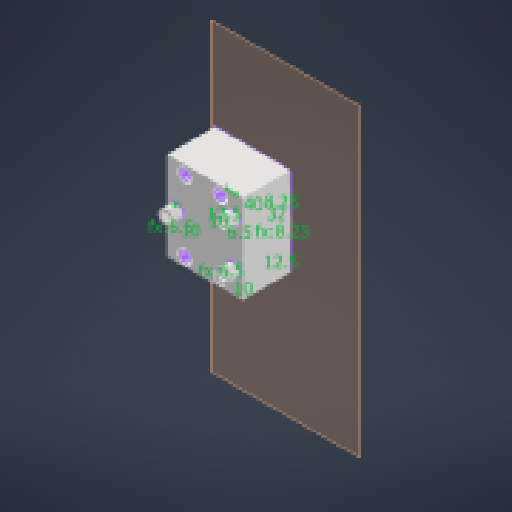
# Autodesk Inventor part: Printer_head_mount
Saved by Autodesk Inventor 2027 (Build 310192060, 192F)
## iProperties
Created: 2026-06-01
Part Number: Printer_head_mount
Material: Generic
Document SubType Name: Modeling
Designer: jacob
Density: 1 g/cm^3
Appearance: Default
Author: jacob
Autodesk Inventor part; units mm, degrees
ref_plane "YZ Plane" through (0, 0, 0) normal (1, 0, 0) x (0, 1, 0)
ref_plane "XZ Plane" through (0, 0, 0) normal (0, 1, 0) x (-1, 0, 0)
ref_plane "XY Plane" through (0, 0, 0) normal (0, 0, 1) x (1, 0, 0)
ref_plane "Work Plane1" through (0, 0, 0) normal (0, 0, 1) x (1, 0, 0)
sketch "base_sketch" plane through (0, 0, 0) normal (0, 0, 1) x (1, 0, 0)
  line L0 (3.4991, 43.75) -> (-50, 43.75)
  line L1 (-50, 43.75) -> (-50, -18.8295)
  line L2 (-50, -18.8295) -> (3.4991, -18.8295)
  line L3 (3.4991, -18.8295) -> (3.4991, 43.75)
  line L4 (-37.5, -12.5795) -> (-37.5, -18.8295)
  line L5 (-37.5, -12.5795) -> (-50, -12.5795)
  line L6 (3.4991, -12.3536) -> (-9, -12.5)
  line L7 (-2.7504, -12.4268) -> (-2.7504, -3.4634)
  line L8 (-2.7504, -3.4634) -> (-2.7504, -11.9897)
  line L9 (-2.7504, 37.5) -> (-2.7504, 28.5366)
  line L10 (-2.791, 23.7736) -> (-6.8956, 26.1903)
  line L11 (-6.8956, 26.1903) -> (-6.855, 30.9533)
  line L12 (-6.855, 30.9533) -> (-2.7098, 33.2996)
  line L13 (-2.7098, 33.2996) -> (1.3947, 30.8829)
  line L14 (1.3947, 30.8829) -> (1.3541, 26.12)
  line L15 (1.3541, 26.12) -> (-2.791, 23.7736)
  line L16 (-2.762, 1.2997) -> (1.3688, -1.0718)
  line L17 (1.3688, -1.0718) -> (1.3804, -5.8349)
  line L18 (1.3804, -5.8349) -> (-2.7388, -8.2265)
  line L19 (-2.7388, -8.2265) -> (-6.8696, -5.855)
  line L20 (-6.8696, -5.855) -> (-6.8812, -1.0919)
  line L21 (-6.8812, -1.0919) -> (-2.762, 1.2997)
  line L22 (-2.7504, 28.5366) -> (-2.7504, -3.4634)
  line L23 (-2.7504, -3.4634) -> (-2.7504, 12.5366)
  line L24 (-2.7504, 12.5366) -> (-42.7504, 12.5366)
  line L25 (-42.7504, 7.7735) -> (-46.8754, 10.155)
  line L26 (-46.8754, 10.155) -> (-46.8754, 14.9182)
  line L27 (-46.8754, 14.9182) -> (-42.7504, 17.2998)
  line L28 (-42.7504, 17.2998) -> (-38.6254, 14.9182)
  line L29 (-38.6254, 14.9182) -> (-38.6254, 10.155)
  line L30 (-38.6254, 10.155) -> (-42.7504, 7.7735)
  dimension "d20" = 12.5
  dimension "d26" = 12.5
  dimension "d29" = 32
  dimension "d30" = 8.25
  dimension "d31" = 8.25
  dimension "d32" = 40
  constraints: 62 end point, 4 perpendicular, 4 point on line, 3 coincident, 3 vertical, 2 midpoint, 2 parallel, 1 collinear, 1 horizontal, 39 other
  measures "d20" distance of L4.start L5.end
  measures "d26" distance of L6.start L6.end
  measures "d29" distance of L7.end L9.end
  measures "d30" distance between parallel lines of L11 L14
  measures "d31" distance between parallel lines of L20 L17
  measures "d32" distance of L23.end L24.end
extrude "first" add sketch "base_sketch" along normal blind 20
sketch "Sketch6" plane through (0, 0, 20) normal (0, 0, 1) x (1, 0, 0)
  line L0 (3.4991, 43.75) -> (-50, 43.75) projected
  line L1 (-50, 43.75) -> (-50, -18.8295) projected
  line L2 (-50, -18.8295) -> (3.4991, -18.8295) projected
  line L3 (3.4991, -18.8295) -> (3.4991, 43.75) projected
  line L4 (-38.6254, 14.9182) -> (-38.6254, 10.155) projected
  line L5 (-38.6254, 10.155) -> (-42.7504, 7.7735) projected
  line L6 (-42.7504, 7.7735) -> (-46.8754, 10.155) projected
  line L7 (-46.8754, 10.155) -> (-46.8754, 14.9182) projected
  line L8 (-46.8754, 14.9182) -> (-42.7504, 17.2998) projected
  line L9 (-42.7504, 17.2998) -> (-38.6254, 14.9182) projected
  line L10 (1.3541, 26.12) -> (-2.791, 23.7736) projected
  line L11 (-2.791, 23.7736) -> (-6.8956, 26.1903) projected
  line L12 (-6.8956, 26.1903) -> (-6.855, 30.9533) projected
  line L13 (-6.855, 30.9533) -> (-2.7098, 33.2996) projected
  line L14 (-2.7098, 33.2996) -> (1.3947, 30.8829) projected
  line L15 (1.3947, 30.8829) -> (1.3541, 26.12) projected
  line L16 (-2.762, 1.2997) -> (1.3688, -1.0718) projected
  line L17 (1.3688, -1.0718) -> (1.3804, -5.8349) projected
  line L18 (1.3804, -5.8349) -> (-2.7388, -8.2265) projected
  line L19 (-2.7388, -8.2265) -> (-6.8696, -5.855) projected
  line L20 (-6.8696, -5.855) -> (-6.8812, -1.0919) projected
  line L21 (-6.8812, -1.0919) -> (-2.762, 1.2997) projected
  circle A0 centre (-12.5, 37.5) radius 3.25 projected
  point P0 (0, 0)
extrude "middle" add sketch "Sketch6" along normal blind 7 from surface at 0
sketch "Sketch7" plane through (0, 0, 27) normal (0, 0, 1) x (1, 0, 0)
  line L0 (-50, 43.75) -> (-50, -18.8295) projected
  line L1 (-50, -18.8295) -> (3.4991, -18.8295) projected
  line L2 (3.4991, -18.8295) -> (3.4991, 43.75) projected
  line L3 (3.4991, 43.75) -> (-50, 43.75) projected
  circle A0 centre (-12.25, -12.5) radius 3.25 projected
  circle A1 centre (-37.5, 37.5) radius 3.25 projected
  circle A2 centre (-37.5, -12.5795) radius 3.25 projected
  point P0 (0, 0)
extrude "top" add sketch "Sketch7" along normal blind 7 contours L3 L2 L1 L0 | A0 | A1 | A2
sketch "standoffs" plane through (0, 0, 34) normal (0, 0, 1) x (1, 0, 0)
  circle A0 centre (-3.0004, 28.5366) radius 3.25
  circle A1 centre (-3.0004, -3.4634) radius 3.25
  circle A2 centre (-43.0004, 12.5366) radius 3.25
  circle A3 centre (-3.0004, 28.5366) radius 5
  circle A4 centre (-3.0004, -3.4634) radius 5
  circle A5 centre (-43.0004, 12.5366) radius 5
  dimension "d54" = 10
  dimension "d55" = 10
  dimension "d56" = 10
  dimension "d61" = 6.5
  dimension "d62" = 6.5
  dimension "d63" = 6.5
  constraints: 6 centre point, 3 coincident
  measures "d54" diameter of A3
  measures "d55" diameter of A4
  measures "d56" diameter of A5
  measures "d61" diameter of A0
  measures "d62" diameter of A1
  measures "d63" diameter of A2
extrude "Extrusion7" add sketch "standoffs" along normal blind 8
sketch "label_sketch" plane through (-50, -18.8295, 0) normal (-1, 0, 0) x (0, 0, 1)
  line L0 (21.8439, 46.335) -> (21.8439, 9.2504) construction
  line L1 (21.8439, 9.2504) -> (5.5419, 9.2504) construction
  line L2 (5.5419, 9.2504) -> (5.5419, 46.335) construction
  line L3 (5.5419, 46.335) -> (21.8439, 46.335) construction
  spline S0 degree 2 poles (20.7892, 44.0996) (20.5916, 44.0996) (20.2359, 44.2404) (20.1124, 44.3664) knots 0 0 0 1 2 2 2
  spline S1 degree 2 poles (20.1124, 44.3664) (19.9568, 44.5244) (19.7963, 44.9518) (19.7963, 45.2778) knots 0 0 0 1 2 2 2
  line L4 (19.7963, 45.2778) -> (19.7963, 45.6211)
  line L5 (19.7963, 45.6211) -> (18.6601, 45.6211)
  line L6 (18.6601, 45.6211) -> (18.6601, 46.0262)
  line L7 (18.6601, 46.0262) -> (21.7081, 46.0262)
  line L8 (21.7081, 46.0262) -> (21.7081, 45.2605)
  spline S2 degree 2 poles (21.7081, 45.2605) (21.7081, 44.9888) (21.6191, 44.6084) (21.5179, 44.4627) knots 0 0 0 1 2 2 2
  spline S3 degree 2 poles (21.5179, 44.4627) (21.4018, 44.2923) (21.0436, 44.0996) (20.7892, 44.0996) knots 0 0 0 1 2 2 2
  spline S4 degree 2 poles (20.7769, 44.522) (20.9349, 44.522) (21.1671, 44.6307) (21.2412, 44.7418) knots 0 0 0 1 2 2 2
  spline S5 degree 2 poles (21.2412, 44.7418) (21.3055, 44.8381) (21.3573, 45.095) (21.3573, 45.2852) knots 0 0 0 1 2 2 2
  line L9 (21.3573, 45.2852) -> (21.3573, 45.6211)
  line L10 (21.3573, 45.6211) -> (20.1421, 45.6211)
  line L11 (20.1421, 45.6211) -> (20.1421, 45.3445)
  spline S6 degree 2 poles (20.1421, 45.3445) (20.1421, 45.0975) (20.2211, 44.7937) (20.3249, 44.6949) knots 0 0 0 1 2 2 2
  spline S7 degree 2 poles (20.3249, 44.6949) (20.4162, 44.6035) (20.6311, 44.522) (20.7769, 44.522) knots 0 0 0 1 2 2 2
  line L12 (20.5348, 42.5311) -> (20.5348, 42.5509)
  spline S8 degree 2 poles (20.5348, 42.5509) (20.5472, 42.5954) (20.5521, 42.6917) (20.5521, 42.7584) knots 0 0 0 1 2 2 2
  spline S9 degree 2 poles (20.5521, 42.7584) (20.5521, 42.914) (20.4162, 43.2203) (20.2829, 43.3586) knots 0 0 0 1 2 2 2
  line L13 (20.2829, 43.3586) -> (18.6601, 43.3586)
  line L14 (18.6601, 43.3586) -> (18.6601, 43.7439)
  line L15 (18.6601, 43.7439) -> (20.9473, 43.7439)
  line L16 (20.9473, 43.7439) -> (20.9473, 43.3586)
  line L17 (20.9473, 43.3586) -> (20.6064, 43.3586)
  spline S10 degree 2 poles (20.6064, 43.3586) (20.7942, 43.1486) (20.9473, 42.835) (20.9473, 42.6868) knots 0 0 0 1 2 2 2
  spline S11 degree 2 poles (20.9473, 42.6868) (20.9473, 42.6275) (20.9424, 42.5682) (20.9349, 42.5311) knots 0 0 0 1 2 2 2
  line L18 (20.9349, 42.5311) -> (20.5348, 42.5311)
  line L19 (18.6601, 41.8395) -> (18.6601, 42.2249)
  line L20 (18.6601, 42.2249) -> (20.9473, 42.2249)
  line L21 (20.9473, 42.2249) -> (20.9473, 41.8395)
  line L22 (20.9473, 41.8395) -> (18.6601, 41.8395)
  line L23 (21.3277, 41.8124) -> (21.3277, 42.2496)
  line L24 (21.3277, 42.2496) -> (21.7278, 42.2496)
  line L25 (21.7278, 42.2496) -> (21.7278, 41.8124)
  line L26 (21.7278, 41.8124) -> (21.3277, 41.8124)
  line L27 (18.6601, 39.4782) -> (18.6601, 39.8635)
  line L28 (18.6601, 39.8635) -> (19.9642, 39.8635)
  spline S12 degree 2 poles (19.9642, 39.8635) (20.1223, 39.8635) (20.394, 39.8932) (20.4755, 39.9376) knots 0 0 0 1 2 2 2
  spline S13 degree 2 poles (20.4755, 39.9376) (20.562, 39.9846) (20.646, 40.1525) (20.646, 40.2958) knots 0 0 0 1 2 2 2
  spline S14 degree 2 poles (20.646, 40.2958) (20.646, 40.439) (20.4928, 40.7428) (20.3693, 40.8886) knots 0 0 0 1 2 2 2
  line L29 (20.3693, 40.8886) -> (18.6601, 40.8886)
  line L30 (18.6601, 40.8886) -> (18.6601, 41.2739)
  line L31 (18.6601, 41.2739) -> (20.9473, 41.2739)
  line L32 (20.9473, 41.2739) -> (20.9473, 40.8886)
  line L33 (20.9473, 40.8886) -> (20.6929, 40.8886)
  spline S15 degree 2 poles (20.6929, 40.8886) (20.8485, 40.7157) (21.0115, 40.3822) (21.0115, 40.1945) knots 0 0 0 1 2 2 2
  spline S16 degree 2 poles (21.0115, 40.1945) (21.0115, 39.8586) (20.5669, 39.4782) (20.1445, 39.4782) knots 0 0 0 1 2 2 2
  line L34 (20.1445, 39.4782) -> (18.6601, 39.4782)
  spline S17 degree 2 poles (18.6156, 38.2457) (18.6156, 38.5594) (18.9738, 38.9126) (19.3615, 38.9126) knots 0 0 0 1 2 2 2
  line L35 (19.3615, 38.9126) -> (20.6287, 38.9126)
  line L36 (20.6287, 38.9126) -> (20.6287, 39.1719)
  line L37 (20.6287, 39.1719) -> (20.9473, 39.1719)
  line L38 (20.9473, 39.1719) -> (20.9473, 38.9126)
  line L39 (20.9473, 38.9126) -> (21.6043, 38.9126)
  line L40 (21.6043, 38.9126) -> (21.6043, 38.5272)
  line L41 (21.6043, 38.5272) -> (20.9473, 38.5272)
  line L42 (20.9473, 38.5272) -> (20.9473, 37.8184)
  line L43 (20.9473, 37.8184) -> (20.6287, 37.8184)
  line L44 (20.6287, 37.8184) -> (20.6287, 38.5272)
  line L45 (20.6287, 38.5272) -> (19.5394, 38.5272)
  spline S18 degree 2 poles (19.5394, 38.5272) (19.3665, 38.5272) (19.1763, 38.5149) (19.0948, 38.4729) knots 0 0 0 1 2 2 2
  spline S19 degree 2 poles (19.0948, 38.4729) (19.0232, 38.4383) (18.9515, 38.2827) (18.9515, 38.1493) knots 0 0 0 1 2 2 2
  spline S20 degree 2 poles (18.9515, 38.1493) (18.9515, 38.0555) (19.0083, 37.8801) (19.0256, 37.8406) knots 0 0 0 1 2 2 2
  line L46 (19.0256, 37.8406) -> (19.0256, 37.8184)
  line L47 (19.0256, 37.8184) -> (18.6798, 37.8184)
  spline S21 degree 2 poles (18.6798, 37.8184) (18.6502, 37.927) (18.6156, 38.1493) (18.6156, 38.2457) knots 0 0 0 1 2 2 2
  spline S22 degree 2 poles (18.6082, 36.5414) (18.6082, 37.0897) (19.2232, 37.6924) (19.7913, 37.6924) knots 0 0 0 1 2 2 2
  spline S23 degree 2 poles (19.7913, 37.6924) (20.3496, 37.6924) (21.0115, 37.107) (21.0115, 36.6352) knots 0 0 0 1 2 2 2
  spline S24 degree 2 poles (21.0115, 36.6352) (21.0115, 36.4228) (20.888, 36.0943) (20.7571, 35.9732) knots 0 0 0 1 2 2 2
  spline S25 degree 2 poles (20.7571, 35.9732) (20.6262, 35.8497) (20.2483, 35.7188) (19.9741, 35.7188) knots 0 0 0 1 2 2 2
  line L48 (19.9741, 35.7188) -> (19.7642, 35.7188)
  line L49 (19.7642, 35.7188) -> (19.7642, 37.3021)
  spline S26 degree 2 poles (19.7642, 37.3021) (19.3665, 37.3021) (18.9441, 36.902) (18.9441, 36.5463) knots 0 0 0 1 2 2 2
  spline S27 degree 2 poles (18.9441, 36.5463) (18.9441, 36.4203) (19.0009, 36.1758) (19.0454, 36.077) knots 0 0 0 1 2 2 2
  spline S28 degree 2 poles (19.0454, 36.077) (19.0948, 35.9732) (19.1812, 35.83) (19.2208, 35.7831) knots 0 0 0 1 2 2 2
  line L50 (19.2208, 35.7831) -> (19.2208, 35.7608)
  line L51 (19.2208, 35.7608) -> (18.8009, 35.7608)
  spline S29 degree 2 poles (18.8009, 35.7608) (18.7737, 35.8275) (18.6946, 36.0301) (18.6724, 36.1091) knots 0 0 0 1 2 2 2
  spline S30 degree 2 poles (18.6724, 36.1091) (18.6403, 36.2203) (18.6082, 36.403) (18.6082, 36.5414) knots 0 0 0 1 2 2 2
  spline S31 degree 2 poles (20.0581, 36.0943) (20.2137, 36.0992) (20.4409, 36.1634) (20.5175, 36.2252) knots 0 0 0 1 2 2 2
  spline S32 degree 2 poles (20.5175, 36.2252) (20.604, 36.2919) (20.6954, 36.5018) (20.6954, 36.6574) knots 0 0 0 1 2 2 2
  spline S33 degree 2 poles (20.6954, 36.6574) (20.6954, 36.8106) (20.604, 37.0255) (20.515, 37.1144) knots 0 0 0 1 2 2 2
  spline S34 degree 2 poles (20.515, 37.1144) (20.4237, 37.2008) (20.2038, 37.2898) (20.0581, 37.3021) knots 0 0 0 1 2 2 2
  line L52 (20.0581, 37.3021) -> (20.0581, 36.0943)
  line L53 (20.5348, 34.1158) -> (20.5348, 34.1356)
  spline S35 degree 2 poles (20.5348, 34.1356) (20.5472, 34.18) (20.5521, 34.2763) (20.5521, 34.343) knots 0 0 0 1 2 2 2
  spline S36 degree 2 poles (20.5521, 34.343) (20.5521, 34.4986) (20.4162, 34.8049) (20.2829, 34.9433) knots 0 0 0 1 2 2 2
  line L54 (20.2829, 34.9433) -> (18.6601, 34.9433)
  line L55 (18.6601, 34.9433) -> (18.6601, 35.3286)
  line L56 (18.6601, 35.3286) -> (20.9473, 35.3286)
  line L57 (20.9473, 35.3286) -> (20.9473, 34.9433)
  line L58 (20.9473, 34.9433) -> (20.6064, 34.9433)
  spline S37 degree 2 poles (20.6064, 34.9433) (20.7942, 34.7333) (20.9473, 34.4196) (20.9473, 34.2714) knots 0 0 0 1 2 2 2
  spline S38 degree 2 poles (20.9473, 34.2714) (20.9473, 34.2121) (20.9424, 34.1528) (20.9349, 34.1158) knots 0 0 0 1 2 2 2
  line L59 (20.9349, 34.1158) -> (20.5348, 34.1158)
  line L60 (18.6601, 32.0212) -> (18.6601, 32.4065)
  line L61 (18.6601, 32.4065) -> (19.9642, 32.4065)
  spline S39 degree 2 poles (19.9642, 32.4065) (20.1223, 32.4065) (20.394, 32.4362) (20.4755, 32.4806) knots 0 0 0 1 2 2 2
  spline S40 degree 2 poles (20.4755, 32.4806) (20.562, 32.5276) (20.646, 32.6955) (20.646, 32.8388) knots 0 0 0 1 2 2 2
  spline S41 degree 2 poles (20.646, 32.8388) (20.646, 32.9821) (20.4928, 33.2859) (20.3693, 33.4316) knots 0 0 0 1 2 2 2
  line L62 (20.3693, 33.4316) -> (18.6601, 33.4316)
  line L63 (18.6601, 33.4316) -> (18.6601, 33.8169)
  line L64 (18.6601, 33.8169) -> (21.8439, 33.8169)
  line L65 (21.8439, 33.8169) -> (21.8439, 33.4316)
  line L66 (21.8439, 33.4316) -> (20.6929, 33.4316)
  spline S42 degree 2 poles (20.6929, 33.4316) (20.8485, 33.2587) (21.0115, 32.9252) (21.0115, 32.7375) knots 0 0 0 1 2 2 2
  spline S43 degree 2 poles (21.0115, 32.7375) (21.0115, 32.4016) (20.5669, 32.0212) (20.1445, 32.0212) knots 0 0 0 1 2 2 2
  line L67 (20.1445, 32.0212) -> (18.6601, 32.0212)
  spline S44 degree 2 poles (18.6082, 30.4873) (18.6082, 31.0357) (19.2232, 31.6384) (19.7913, 31.6384) knots 0 0 0 1 2 2 2
  spline S45 degree 2 poles (19.7913, 31.6384) (20.3496, 31.6384) (21.0115, 31.053) (21.0115, 30.5812) knots 0 0 0 1 2 2 2
  spline S46 degree 2 poles (21.0115, 30.5812) (21.0115, 30.3688) (20.888, 30.0403) (20.7571, 29.9192) knots 0 0 0 1 2 2 2
  spline S47 degree 2 poles (20.7571, 29.9192) (20.6262, 29.7957) (20.2483, 29.6648) (19.9741, 29.6648) knots 0 0 0 1 2 2 2
  line L68 (19.9741, 29.6648) -> (19.7642, 29.6648)
  line L69 (19.7642, 29.6648) -> (19.7642, 31.2481)
  spline S48 degree 2 poles (19.7642, 31.2481) (19.3665, 31.2481) (18.9441, 30.848) (18.9441, 30.4923) knots 0 0 0 1 2 2 2
  spline S49 degree 2 poles (18.9441, 30.4923) (18.9441, 30.3663) (19.0009, 30.1218) (19.0454, 30.023) knots 0 0 0 1 2 2 2
  spline S50 degree 2 poles (19.0454, 30.023) (19.0948, 29.9192) (19.1812, 29.776) (19.2208, 29.729) knots 0 0 0 1 2 2 2
  line L70 (19.2208, 29.729) -> (19.2208, 29.7068)
  line L71 (19.2208, 29.7068) -> (18.8009, 29.7068)
  spline S51 degree 2 poles (18.8009, 29.7068) (18.7737, 29.7735) (18.6946, 29.976) (18.6724, 30.0551) knots 0 0 0 1 2 2 2
  spline S52 degree 2 poles (18.6724, 30.0551) (18.6403, 30.1662) (18.6082, 30.349) (18.6082, 30.4873) knots 0 0 0 1 2 2 2
  spline S53 degree 2 poles (20.0581, 30.0403) (20.2137, 30.0452) (20.4409, 30.1094) (20.5175, 30.1712) knots 0 0 0 1 2 2 2
  spline S54 degree 2 poles (20.5175, 30.1712) (20.604, 30.2379) (20.6954, 30.4478) (20.6954, 30.6034) knots 0 0 0 1 2 2 2
  spline S55 degree 2 poles (20.6954, 30.6034) (20.6954, 30.7566) (20.604, 30.9715) (20.515, 31.0604) knots 0 0 0 1 2 2 2
  spline S56 degree 2 poles (20.515, 31.0604) (20.4237, 31.1468) (20.2038, 31.2358) (20.0581, 31.2481) knots 0 0 0 1 2 2 2
  line L72 (20.0581, 31.2481) -> (20.0581, 30.0403)
  spline S57 degree 2 poles (18.9021, 28) (18.8675, 28.047) (18.744, 28.205) (18.707, 28.2791) knots 0 0 0 1 2 2 2
  spline S58 degree 2 poles (18.707, 28.2791) (18.6527, 28.3804) (18.5958, 28.5706) (18.5958, 28.7435) knots 0 0 0 1 2 2 2
  spline S59 degree 2 poles (18.5958, 28.7435) (18.5958, 28.8843) (18.7021, 29.1387) (18.7984, 29.235) knots 0 0 0 1 2 2 2
  spline S60 degree 2 poles (18.7984, 29.235) (18.8922, 29.3264) (19.1689, 29.4376) (19.322, 29.4376) knots 0 0 0 1 2 2 2
  spline S61 degree 2 poles (19.322, 29.4376) (19.5591, 29.4376) (19.8951, 29.2375) (19.9914, 29.0202) knots 0 0 0 1 2 2 2
  spline S62 degree 2 poles (19.9914, 29.0202) (20.0803, 28.8275) (20.147, 28.3038) (20.1643, 28) knots 0 0 0 1 2 2 2
  line L73 (20.1643, 28) -> (20.2384, 28)
  spline S63 degree 2 poles (20.2384, 28) (20.3718, 28) (20.5373, 28.0815) (20.5842, 28.1556) knots 0 0 0 1 2 2 2
  spline S64 degree 2 poles (20.5842, 28.1556) (20.6311, 28.2297) (20.6608, 28.4422) (20.6608, 28.5558) knots 0 0 0 1 2 2 2
  spline S65 degree 2 poles (20.6608, 28.5558) (20.6608, 28.6892) (20.5817, 29.0498) (20.5052, 29.2301) knots 0 0 0 1 2 2 2
  line L74 (20.5052, 29.2301) -> (20.5052, 29.2523)
  line L75 (20.5052, 29.2523) -> (20.8979, 29.2523)
  spline S66 degree 2 poles (20.8979, 29.2523) (20.9275, 29.1461) (21.0016, 28.7485) (21.0016, 28.5533) knots 0 0 0 1 2 2 2
  spline S67 degree 2 poles (21.0016, 28.5533) (21.0016, 28.3162) (20.9275, 27.9926) (20.8312, 27.8642) knots 0 0 0 1 2 2 2
  spline S68 degree 2 poles (20.8312, 27.8642) (20.7373, 27.7382) (20.4385, 27.6147) (20.2236, 27.6147) knots 0 0 0 1 2 2 2
  line L76 (20.2236, 27.6147) -> (18.6601, 27.6147)
  line L77 (18.6601, 27.6147) -> (18.6601, 28)
  line L78 (18.6601, 28) -> (18.9021, 28)
  line L79 (19.2232, 28) -> (19.858, 28)
  spline S69 degree 2 poles (19.858, 28) (19.8457, 28.1384) (19.8037, 28.5558) (19.7642, 28.6867) knots 0 0 0 1 2 2 2
  spline S70 degree 2 poles (19.7642, 28.6867) (19.7172, 28.8398) (19.5221, 29.0399) (19.3492, 29.0399) knots 0 0 0 1 2 2 2
  spline S71 degree 2 poles (19.3492, 29.0399) (19.1516, 29.0399) (18.9515, 28.8176) (18.9515, 28.6052) knots 0 0 0 1 2 2 2
  spline S72 degree 2 poles (18.9515, 28.6052) (18.9515, 28.4249) (19.1071, 28.1285) (19.2232, 28) knots 0 0 0 1 2 2 2
  line L80 (18.6601, 25.3151) -> (18.6601, 25.7005)
  line L81 (18.6601, 25.7005) -> (18.8922, 25.7005)
  spline S73 degree 2 poles (18.8922, 25.7005) (18.8181, 25.7894) (18.7193, 25.9203) (18.6774, 26.0092) knots 0 0 0 1 2 2 2
  spline S74 degree 2 poles (18.6774, 26.0092) (18.6378, 26.0907) (18.5958, 26.2661) (18.5958, 26.3822) knots 0 0 0 1 2 2 2
  spline S75 degree 2 poles (18.5958, 26.3822) (18.5958, 26.5699) (18.7515, 26.8861) (18.9021, 26.9972) knots 0 0 0 1 2 2 2
  spline S76 degree 2 poles (18.9021, 26.9972) (19.0528, 27.1084) (19.4974, 27.2319) (19.7864, 27.2319) knots 0 0 0 1 2 2 2
  spline S77 degree 2 poles (19.7864, 27.2319) (20.0877, 27.2319) (20.5274, 27.0763) (20.6929, 26.9404) knots 0 0 0 1 2 2 2
  spline S78 degree 2 poles (20.6929, 26.9404) (20.8411, 26.8144) (21.0115, 26.4612) (21.0115, 26.2661) knots 0 0 0 1 2 2 2
  spline S79 degree 2 poles (21.0115, 26.2661) (21.0115, 26.0957) (20.9349, 25.8412) (20.8559, 25.7005) knots 0 0 0 1 2 2 2
  line L82 (20.8559, 25.7005) -> (21.8439, 25.7005)
  line L83 (21.8439, 25.7005) -> (21.8439, 25.3151)
  line L84 (21.8439, 25.3151) -> (18.6601, 25.3151)
  line L85 (19.2158, 25.7005) -> (20.5373, 25.7005)
  spline S80 degree 2 poles (20.5373, 25.7005) (20.6064, 25.8437) (20.6583, 26.071) (20.6583, 26.2019) knots 0 0 0 1 2 2 2
  spline S81 degree 2 poles (20.6583, 26.2019) (20.6583, 26.4983) (20.2137, 26.8342) (19.7938, 26.8342) knots 0 0 0 1 2 2 2
  spline S82 degree 2 poles (19.7938, 26.8342) (19.3887, 26.8342) (18.9614, 26.5773) (18.9614, 26.2933) knots 0 0 0 1 2 2 2
  spline S83 degree 2 poles (18.9614, 26.2933) (18.9614, 26.1426) (19.0997, 25.8363) (19.2158, 25.7005) knots 0 0 0 1 2 2 2
  line L86 (18.6601, 20.8543) -> (19.984, 20.8543)
  spline S84 degree 2 poles (19.984, 20.8543) (20.1421, 20.8543) (20.4113, 20.879) (20.4854, 20.9185) knots 0 0 0 1 2 2 2
  spline S85 degree 2 poles (20.4854, 20.9185) (20.5669, 20.958) (20.646, 21.1087) (20.646, 21.2396) knots 0 0 0 1 2 2 2
  spline S86 degree 2 poles (20.646, 21.2396) (20.646, 21.3582) (20.5002, 21.6299) (20.3619, 21.7731) knots 0 0 0 1 2 2 2
  spline S87 degree 2 poles (20.3619, 21.7731) (20.3273, 21.7707) (20.231, 21.7657) (20.1668, 21.7657) knots 0 0 0 1 2 2 2
  line L87 (20.1668, 21.7657) -> (18.6601, 21.7657)
  line L88 (18.6601, 21.7657) -> (18.6601, 22.151)
  line L89 (18.6601, 22.151) -> (19.984, 22.151)
  spline S88 degree 2 poles (19.984, 22.151) (20.1421, 22.151) (20.4113, 22.1757) (20.4854, 22.2153) knots 0 0 0 1 2 2 2
  spline S89 degree 2 poles (20.4854, 22.2153) (20.5669, 22.2548) (20.646, 22.4054) (20.646, 22.5364) knots 0 0 0 1 2 2 2
  spline S90 degree 2 poles (20.646, 22.5364) (20.646, 22.6599) (20.4903, 22.934) (20.3693, 23.0625) knots 0 0 0 1 2 2 2
  line L90 (20.3693, 23.0625) -> (18.6601, 23.0625)
  line L91 (18.6601, 23.0625) -> (18.6601, 23.4478)
  line L92 (18.6601, 23.4478) -> (20.9473, 23.4478)
  line L93 (20.9473, 23.4478) -> (20.9473, 23.0625)
  line L94 (20.9473, 23.0625) -> (20.6954, 23.0625)
  spline S91 degree 2 poles (20.6954, 23.0625) (20.846, 22.9118) (21.0115, 22.6154) (21.0115, 22.4376) knots 0 0 0 1 2 2 2
  spline S92 degree 2 poles (21.0115, 22.4376) (21.0115, 22.235) (20.8263, 21.9213) (20.6163, 21.8398) knots 0 0 0 1 2 2 2
  spline S93 degree 2 poles (20.6163, 21.8398) (20.8114, 21.6644) (21.0115, 21.3335) (21.0115, 21.1408) knots 0 0 0 1 2 2 2
  spline S94 degree 2 poles (21.0115, 21.1408) (21.0115, 20.9926) (20.9201, 20.7505) (20.8164, 20.6616) knots 0 0 0 1 2 2 2
  spline S95 degree 2 poles (20.8164, 20.6616) (20.7126, 20.5702) (20.4014, 20.469) (20.1668, 20.469) knots 0 0 0 1 2 2 2
  line L95 (20.1668, 20.469) -> (18.6601, 20.469)
  line L96 (18.6601, 20.469) -> (18.6601, 20.8543)
  spline S96 degree 2 poles (19.8037, 18.0483) (19.2257, 18.0483) (18.5958, 18.6041) (18.5958, 19.0685) knots 0 0 0 1 2 2 2
  spline S97 degree 2 poles (18.5958, 19.0685) (18.5958, 19.5452) (19.2455, 20.091) (19.8037, 20.091) knots 0 0 0 1 2 2 2
  spline S98 degree 2 poles (19.8037, 20.091) (20.3767, 20.091) (21.0115, 19.5279) (21.0115, 19.0685) knots 0 0 0 1 2 2 2
  spline S99 degree 2 poles (21.0115, 19.0685) (21.0115, 18.6041) (20.3792, 18.0483) (19.8037, 18.0483) knots 0 0 0 1 2 2 2
  spline S100 degree 2 poles (19.8037, 18.446) (20.2483, 18.446) (20.6805, 18.7696) (20.6805, 19.0685) knots 0 0 0 1 2 2 2
  spline S101 degree 2 poles (20.6805, 19.0685) (20.6805, 19.3673) (20.2483, 19.6934) (19.8037, 19.6934) knots 0 0 0 1 2 2 2
  spline S102 degree 2 poles (19.8037, 19.6934) (19.3714, 19.6934) (18.9268, 19.3673) (18.9268, 19.0685) knots 0 0 0 1 2 2 2
  spline S103 degree 2 poles (18.9268, 19.0685) (18.9268, 18.7721) (19.364, 18.446) (19.8037, 18.446) knots 0 0 0 1 2 2 2
  line L97 (18.6601, 15.8747) -> (18.6601, 16.26)
  line L98 (18.6601, 16.26) -> (18.912, 16.26)
  spline S104 degree 2 poles (18.912, 16.26) (18.7564, 16.4379) (18.5958, 16.7565) (18.5958, 16.9541) knots 0 0 0 1 2 2 2
  spline S105 degree 2 poles (18.5958, 16.9541) (18.5958, 17.1023) (18.6946, 17.3666) (18.8009, 17.4629) knots 0 0 0 1 2 2 2
  spline S106 degree 2 poles (18.8009, 17.4629) (18.9071, 17.5617) (19.2306, 17.6704) (19.4628, 17.6704) knots 0 0 0 1 2 2 2
  line L99 (19.4628, 17.6704) -> (20.9473, 17.6704)
  line L100 (20.9473, 17.6704) -> (20.9473, 17.2851)
  line L101 (20.9473, 17.2851) -> (19.6431, 17.2851)
  spline S107 degree 2 poles (19.6431, 17.2851) (19.4603, 17.2851) (19.2208, 17.2579) (19.1318, 17.211) knots 0 0 0 1 2 2 2
  spline S108 degree 2 poles (19.1318, 17.211) (19.0429, 17.1641) (18.9614, 17.0035) (18.9614, 16.8529) knots 0 0 0 1 2 2 2
  spline S109 degree 2 poles (18.9614, 16.8529) (18.9614, 16.7121) (19.122, 16.3934) (19.238, 16.26) knots 0 0 0 1 2 2 2
  line L102 (19.238, 16.26) -> (20.9473, 16.26)
  line L103 (20.9473, 16.26) -> (20.9473, 15.8747)
  line L104 (20.9473, 15.8747) -> (18.6601, 15.8747)
  line L105 (18.6601, 13.5208) -> (18.6601, 13.9061)
  line L106 (18.6601, 13.9061) -> (19.9642, 13.9061)
  spline S110 degree 2 poles (19.9642, 13.9061) (20.1223, 13.9061) (20.394, 13.9358) (20.4755, 13.9802) knots 0 0 0 1 2 2 2
  spline S111 degree 2 poles (20.4755, 13.9802) (20.562, 14.0272) (20.646, 14.1951) (20.646, 14.3384) knots 0 0 0 1 2 2 2
  spline S112 degree 2 poles (20.646, 14.3384) (20.646, 14.4816) (20.4928, 14.7854) (20.3693, 14.9312) knots 0 0 0 1 2 2 2
  line L107 (20.3693, 14.9312) -> (18.6601, 14.9312)
  line L108 (18.6601, 14.9312) -> (18.6601, 15.3165)
  line L109 (18.6601, 15.3165) -> (20.9473, 15.3165)
  line L110 (20.9473, 15.3165) -> (20.9473, 14.9312)
  line L111 (20.9473, 14.9312) -> (20.6929, 14.9312)
  spline S113 degree 2 poles (20.6929, 14.9312) (20.8485, 14.7583) (21.0115, 14.4248) (21.0115, 14.2371) knots 0 0 0 1 2 2 2
  spline S114 degree 2 poles (21.0115, 14.2371) (21.0115, 13.9012) (20.5669, 13.5208) (20.1445, 13.5208) knots 0 0 0 1 2 2 2
  line L112 (20.1445, 13.5208) -> (18.6601, 13.5208)
  spline S115 degree 2 poles (18.6156, 12.2883) (18.6156, 12.602) (18.9738, 12.9552) (19.3615, 12.9552) knots 0 0 0 1 2 2 2
  line L113 (19.3615, 12.9552) -> (20.6287, 12.9552)
  line L114 (20.6287, 12.9552) -> (20.6287, 13.2145)
  line L115 (20.6287, 13.2145) -> (20.9473, 13.2145)
  line L116 (20.9473, 13.2145) -> (20.9473, 12.9552)
  line L117 (20.9473, 12.9552) -> (21.6043, 12.9552)
  line L118 (21.6043, 12.9552) -> (21.6043, 12.5698)
  line L119 (21.6043, 12.5698) -> (20.9473, 12.5698)
  line L120 (20.9473, 12.5698) -> (20.9473, 11.861)
  line L121 (20.9473, 11.861) -> (20.6287, 11.861)
  line L122 (20.6287, 11.861) -> (20.6287, 12.5698)
  line L123 (20.6287, 12.5698) -> (19.5394, 12.5698)
  spline S116 degree 2 poles (19.5394, 12.5698) (19.3665, 12.5698) (19.1763, 12.5575) (19.0948, 12.5155) knots 0 0 0 1 2 2 2
  spline S117 degree 2 poles (19.0948, 12.5155) (19.0232, 12.4809) (18.9515, 12.3253) (18.9515, 12.1919) knots 0 0 0 1 2 2 2
  spline S118 degree 2 poles (18.9515, 12.1919) (18.9515, 12.0981) (19.0083, 11.9227) (19.0256, 11.8832) knots 0 0 0 1 2 2 2
  line L124 (19.0256, 11.8832) -> (19.0256, 11.861)
  line L125 (19.0256, 11.861) -> (18.6798, 11.861)
  spline S119 degree 2 poles (18.6798, 11.861) (18.6502, 11.9696) (18.6156, 12.1919) (18.6156, 12.2883) knots 0 0 0 1 2 2 2
  spline S120 degree 2 poles (14.6296, 44.1861) (14.395, 44.1861) (13.9973, 44.3417) (13.8639, 44.4726) knots 0 0 0 1 2 2 2
  spline S121 degree 2 poles (13.8639, 44.4726) (13.7231, 44.6084) (13.5774, 44.9493) (13.5774, 45.1543) knots 0 0 0 1 2 2 2
  spline S122 degree 2 poles (13.5774, 45.1543) (13.5774, 45.3593) (13.7157, 45.6977) (13.854, 45.8261) knots 0 0 0 1 2 2 2
  spline S123 degree 2 poles (13.854, 45.8261) (14.0195, 45.9842) (14.5753, 46.1621) (14.9804, 46.1621) knots 0 0 0 1 2 2 2
  spline S124 degree 2 poles (14.9804, 46.1621) (15.378, 46.1621) (16.0178, 45.999) (16.2549, 45.8286) knots 0 0 0 1 2 2 2
  spline S125 degree 2 poles (16.2549, 45.8286) (16.4871, 45.6631) (16.7464, 45.1395) (16.7464, 44.7961) knots 0 0 0 1 2 2 2
  spline S126 degree 2 poles (16.7464, 44.7961) (16.7464, 44.6949) (16.7267, 44.517) (16.7044, 44.4503) knots 0 0 0 1 2 2 2
  line L126 (16.7044, 44.4503) -> (16.3117, 44.4503)
  line L127 (16.3117, 44.4503) -> (16.3117, 44.4676)
  spline S127 degree 2 poles (16.3117, 44.4676) (16.3413, 44.5244) (16.3932, 44.7319) (16.3932, 44.8505) knots 0 0 0 1 2 2 2
  spline S128 degree 2 poles (16.3932, 44.8505) (16.3932, 45.2309) (15.8794, 45.6977) (15.3756, 45.7422) knots 0 0 0 1 2 2 2
  spline S129 degree 2 poles (15.3756, 45.7422) (15.4768, 45.5964) (15.588, 45.2901) (15.588, 45.1074) knots 0 0 0 1 2 2 2
  spline S130 degree 2 poles (15.588, 45.1074) (15.588, 44.9295) (15.5164, 44.6628) (15.4077, 44.517) knots 0 0 0 1 2 2 2
  spline S131 degree 2 poles (15.4077, 44.517) (15.2817, 44.3491) (14.8914, 44.1861) (14.6296, 44.1861) knots 0 0 0 1 2 2 2
  spline S132 degree 2 poles (14.6123, 44.601) (14.8, 44.601) (15.0545, 44.6998) (15.1434, 44.8085) knots 0 0 0 1 2 2 2
  spline S133 degree 2 poles (15.1434, 44.8085) (15.2076, 44.89) (15.2496, 45.0925) (15.2496, 45.1988) knots 0 0 0 1 2 2 2
  spline S134 degree 2 poles (15.2496, 45.1988) (15.2496, 45.342) (15.1631, 45.6113) (15.0816, 45.7422) knots 0 0 0 1 2 2 2
  spline S135 degree 2 poles (15.0816, 45.7422) (15.0372, 45.7446) (14.9532, 45.7496) (14.889, 45.7496) knots 0 0 0 1 2 2 2
  spline S136 degree 2 poles (14.889, 45.7496) (14.5728, 45.7496) (14.185, 45.6261) (14.0837, 45.5322) knots 0 0 0 1 2 2 2
  spline S137 degree 2 poles (14.0837, 45.5322) (13.9874, 45.4458) (13.9108, 45.258) (13.9108, 45.1518) knots 0 0 0 1 2 2 2
  spline S138 degree 2 poles (13.9108, 45.1518) (13.9108, 44.9048) (14.2616, 44.601) (14.6123, 44.601) knots 0 0 0 1 2 2 2
  line L128 (16.8255, 42.5583) -> (12.9796, 43.7513)
  line L129 (12.9796, 43.7513) -> (12.9796, 44.0971)
  line L130 (12.9796, 44.0971) -> (16.8255, 42.9091)
  line L131 (16.8255, 42.9091) -> (16.8255, 42.5583)
  line L132 (13.6416, 40.3427) -> (13.6416, 42.2224)
  line L133 (13.6416, 42.2224) -> (14.0739, 42.2224)
  spline S139 degree 2 poles (14.0739, 42.2224) (14.2641, 42.0198) (14.6173, 41.6592) (14.8075, 41.4863) knots 0 0 0 1 2 2 2
  spline S140 degree 2 poles (14.8075, 41.4863) (15.1903, 41.1381) (15.6497, 40.8836) (15.8943, 40.8836) knots 0 0 0 1 2 2 2
  spline S141 degree 2 poles (15.8943, 40.8836) (16.0227, 40.8836) (16.2154, 40.9627) (16.2771, 41.0343) knots 0 0 0 1 2 2 2
  spline S142 degree 2 poles (16.2771, 41.0343) (16.3389, 41.1059) (16.4006, 41.2937) (16.4006, 41.4073) knots 0 0 0 1 2 2 2
  spline S143 degree 2 poles (16.4006, 41.4073) (16.4006, 41.516) (16.3463, 41.7383) (16.3043, 41.8395) knots 0 0 0 1 2 2 2
  spline S144 degree 2 poles (16.3043, 41.8395) (16.2697, 41.926) (16.1709, 42.0865) (16.1363, 42.1359) knots 0 0 0 1 2 2 2
  line L134 (16.1363, 42.1359) -> (16.1363, 42.1582)
  line L135 (16.1363, 42.1582) -> (16.5711, 42.1582)
  spline S145 degree 2 poles (16.5711, 42.1582) (16.6328, 42.0322) (16.7538, 41.5802) (16.7538, 41.3776) knots 0 0 0 1 2 2 2
  spline S146 degree 2 poles (16.7538, 41.3776) (16.7538, 40.9503) (16.3018, 40.4687) (15.9165, 40.4687) knots 0 0 0 1 2 2 2
  spline S147 degree 2 poles (15.9165, 40.4687) (15.7362, 40.4687) (15.4348, 40.5527) (15.3064, 40.6268) knots 0 0 0 1 2 2 2
  spline S148 degree 2 poles (15.3064, 40.6268) (15.173, 40.7009) (14.9112, 40.9158) (14.7852, 41.0343) knots 0 0 0 1 2 2 2
  spline S149 degree 2 poles (14.7852, 41.0343) (14.5753, 41.227) (14.1257, 41.6987) (13.9948, 41.8395) knots 0 0 0 1 2 2 2
  line L136 (13.9948, 41.8395) -> (13.9948, 40.3427)
  line L137 (13.9948, 40.3427) -> (13.6416, 40.3427)
  line L138 (14.6889, 37.974) -> (14.6889, 38.3371)
  line L139 (14.6889, 38.3371) -> (13.6416, 38.3371)
  line L140 (13.6416, 38.3371) -> (13.6416, 38.7298)
  line L141 (13.6416, 38.7298) -> (14.6889, 38.7298)
  line L142 (14.6889, 38.7298) -> (14.6889, 40.0759)
  line L143 (14.6889, 40.0759) -> (15.1187, 40.0759)
  line L144 (15.1187, 40.0759) -> (16.6896, 38.7125)
  line L145 (16.6896, 38.7125) -> (16.6896, 38.3371)
  line L146 (16.6896, 38.3371) -> (15.0174, 38.3371)
  line L147 (15.0174, 38.3371) -> (15.0174, 37.974)
  line L148 (15.0174, 37.974) -> (14.6889, 37.974)
  line L149 (15.0174, 38.7298) -> (16.208, 38.7298)
  line L150 (16.208, 38.7298) -> (15.0174, 39.7548)
  line L151 (15.0174, 39.7548) -> (15.0174, 38.7298)
  line L152 (16.8255, 36.3808) -> (12.9796, 37.5738)
  line L153 (12.9796, 37.5738) -> (12.9796, 37.9196)
  line L154 (12.9796, 37.9196) -> (16.8255, 36.7315)
  line L155 (16.8255, 36.7315) -> (16.8255, 36.3808)
  line L156 (13.6416, 34.1652) -> (13.6416, 36.0449)
  line L157 (13.6416, 36.0449) -> (14.0739, 36.0449)
  spline S150 degree 2 poles (14.0739, 36.0449) (14.2641, 35.8423) (14.6173, 35.4817) (14.8075, 35.3088) knots 0 0 0 1 2 2 2
  spline S151 degree 2 poles (14.8075, 35.3088) (15.1903, 34.9605) (15.6497, 34.7061) (15.8943, 34.7061) knots 0 0 0 1 2 2 2
  spline S152 degree 2 poles (15.8943, 34.7061) (16.0227, 34.7061) (16.2154, 34.7852) (16.2771, 34.8568) knots 0 0 0 1 2 2 2
  spline S153 degree 2 poles (16.2771, 34.8568) (16.3389, 34.9284) (16.4006, 35.1162) (16.4006, 35.2298) knots 0 0 0 1 2 2 2
  spline S154 degree 2 poles (16.4006, 35.2298) (16.4006, 35.3385) (16.3463, 35.5608) (16.3043, 35.662) knots 0 0 0 1 2 2 2
  spline S155 degree 2 poles (16.3043, 35.662) (16.2697, 35.7485) (16.1709, 35.909) (16.1363, 35.9584) knots 0 0 0 1 2 2 2
  line L158 (16.1363, 35.9584) -> (16.1363, 35.9807)
  line L159 (16.1363, 35.9807) -> (16.5711, 35.9807)
  spline S156 degree 2 poles (16.5711, 35.9807) (16.6328, 35.8547) (16.7538, 35.4027) (16.7538, 35.2001) knots 0 0 0 1 2 2 2
  spline S157 degree 2 poles (16.7538, 35.2001) (16.7538, 34.7728) (16.3018, 34.2912) (15.9165, 34.2912) knots 0 0 0 1 2 2 2
  spline S158 degree 2 poles (15.9165, 34.2912) (15.7362, 34.2912) (15.4348, 34.3751) (15.3064, 34.4492) knots 0 0 0 1 2 2 2
  spline S159 degree 2 poles (15.3064, 34.4492) (15.173, 34.5233) (14.9112, 34.7382) (14.7852, 34.8568) knots 0 0 0 1 2 2 2
  spline S160 degree 2 poles (14.7852, 34.8568) (14.5753, 35.0495) (14.1257, 35.5212) (13.9948, 35.662) knots 0 0 0 1 2 2 2
  line L160 (13.9948, 35.662) -> (13.9948, 34.1652)
  line L161 (13.9948, 34.1652) -> (13.6416, 34.1652)
  spline S161 degree 2 poles (15.1656, 31.8607) (14.3456, 31.8607) (13.5774, 32.3374) (13.5774, 32.8339) knots 0 0 0 1 2 2 2
  spline S162 degree 2 poles (13.5774, 32.8339) (13.5774, 33.3377) (14.3604, 33.8095) (15.1631, 33.8095) knots 0 0 0 1 2 2 2
  spline S163 degree 2 poles (15.1631, 33.8095) (15.9881, 33.8095) (16.7514, 33.3328) (16.7514, 32.8339) knots 0 0 0 1 2 2 2
  spline S164 degree 2 poles (16.7514, 32.8339) (16.7514, 32.3324) (15.961, 31.8607) (15.1656, 31.8607) knots 0 0 0 1 2 2 2
  spline S165 degree 2 poles (14.2369, 32.3843) (14.3876, 32.325) (14.8519, 32.2756) (15.1656, 32.2756) knots 0 0 0 1 2 2 2
  spline S166 degree 2 poles (15.1656, 32.2756) (15.4793, 32.2756) (15.9412, 32.325) (16.0968, 32.3868) knots 0 0 0 1 2 2 2
  spline S167 degree 2 poles (16.0968, 32.3868) (16.2524, 32.4485) (16.413, 32.6634) (16.413, 32.8339) knots 0 0 0 1 2 2 2
  spline S168 degree 2 poles (16.413, 32.8339) (16.413, 33.0043) (16.2524, 33.2241) (16.0919, 33.2883) knots 0 0 0 1 2 2 2
  spline S169 degree 2 poles (16.0919, 33.2883) (15.9363, 33.3501) (15.462, 33.3946) (15.1631, 33.3946) knots 0 0 0 1 2 2 2
  spline S170 degree 2 poles (15.1631, 33.3946) (14.842, 33.3946) (14.4123, 33.355) (14.2443, 33.2908) knots 0 0 0 1 2 2 2
  spline S171 degree 2 poles (14.2443, 33.2908) (14.0862, 33.2315) (13.9158, 33.0117) (13.9158, 32.8339) knots 0 0 0 1 2 2 2
  spline S172 degree 2 poles (13.9158, 32.8339) (13.9158, 32.6659) (14.0763, 32.4461) (14.2369, 32.3843) knots 0 0 0 1 2 2 2
  line L162 (13.6416, 29.5907) -> (13.6416, 31.4704)
  line L163 (13.6416, 31.4704) -> (14.0739, 31.4704)
  spline S173 degree 2 poles (14.0739, 31.4704) (14.2641, 31.2679) (14.6173, 30.9072) (14.8075, 30.7343) knots 0 0 0 1 2 2 2
  spline S174 degree 2 poles (14.8075, 30.7343) (15.1903, 30.3861) (15.6497, 30.1317) (15.8943, 30.1317) knots 0 0 0 1 2 2 2
  spline S175 degree 2 poles (15.8943, 30.1317) (16.0227, 30.1317) (16.2154, 30.2107) (16.2771, 30.2823) knots 0 0 0 1 2 2 2
  spline S176 degree 2 poles (16.2771, 30.2823) (16.3389, 30.354) (16.4006, 30.5417) (16.4006, 30.6553) knots 0 0 0 1 2 2 2
  spline S177 degree 2 poles (16.4006, 30.6553) (16.4006, 30.764) (16.3463, 30.9863) (16.3043, 31.0876) knots 0 0 0 1 2 2 2
  spline S178 degree 2 poles (16.3043, 31.0876) (16.2697, 31.174) (16.1709, 31.3346) (16.1363, 31.384) knots 0 0 0 1 2 2 2
  line L164 (16.1363, 31.384) -> (16.1363, 31.4062)
  line L165 (16.1363, 31.4062) -> (16.5711, 31.4062)
  spline S179 degree 2 poles (16.5711, 31.4062) (16.6328, 31.2802) (16.7538, 30.8282) (16.7538, 30.6257) knots 0 0 0 1 2 2 2
  spline S180 degree 2 poles (16.7538, 30.6257) (16.7538, 30.1984) (16.3018, 29.7167) (15.9165, 29.7167) knots 0 0 0 1 2 2 2
  spline S181 degree 2 poles (15.9165, 29.7167) (15.7362, 29.7167) (15.4348, 29.8007) (15.3064, 29.8748) knots 0 0 0 1 2 2 2
  spline S182 degree 2 poles (15.3064, 29.8748) (15.173, 29.9489) (14.9112, 30.1638) (14.7852, 30.2823) knots 0 0 0 1 2 2 2
  spline S183 degree 2 poles (14.7852, 30.2823) (14.5753, 30.475) (14.1257, 30.9468) (13.9948, 31.0876) knots 0 0 0 1 2 2 2
  line L166 (13.9948, 31.0876) -> (13.9948, 29.5907)
  line L167 (13.9948, 29.5907) -> (13.6416, 29.5907)
  spline S184 degree 2 poles (14.6296, 27.2566) (14.395, 27.2566) (13.9973, 27.4122) (13.8639, 27.5431) knots 0 0 0 1 2 2 2
  spline S185 degree 2 poles (13.8639, 27.5431) (13.7231, 27.6789) (13.5774, 28.0198) (13.5774, 28.2248) knots 0 0 0 1 2 2 2
  spline S186 degree 2 poles (13.5774, 28.2248) (13.5774, 28.4298) (13.7157, 28.7682) (13.854, 28.8967) knots 0 0 0 1 2 2 2
  spline S187 degree 2 poles (13.854, 28.8967) (14.0195, 29.0547) (14.5753, 29.2326) (14.9804, 29.2326) knots 0 0 0 1 2 2 2
  spline S188 degree 2 poles (14.9804, 29.2326) (15.378, 29.2326) (16.0178, 29.0696) (16.2549, 28.8991) knots 0 0 0 1 2 2 2
  spline S189 degree 2 poles (16.2549, 28.8991) (16.4871, 28.7336) (16.7464, 28.21) (16.7464, 27.8667) knots 0 0 0 1 2 2 2
  spline S190 degree 2 poles (16.7464, 27.8667) (16.7464, 27.7654) (16.7267, 27.5875) (16.7044, 27.5209) knots 0 0 0 1 2 2 2
  line L168 (16.7044, 27.5209) -> (16.3117, 27.5209)
  line L169 (16.3117, 27.5209) -> (16.3117, 27.5381)
  spline S191 degree 2 poles (16.3117, 27.5381) (16.3413, 27.595) (16.3932, 27.8024) (16.3932, 27.921) knots 0 0 0 1 2 2 2
  spline S192 degree 2 poles (16.3932, 27.921) (16.3932, 28.3014) (15.8794, 28.7682) (15.3756, 28.8127) knots 0 0 0 1 2 2 2
  spline S193 degree 2 poles (15.3756, 28.8127) (15.4768, 28.6669) (15.588, 28.3607) (15.588, 28.1779) knots 0 0 0 1 2 2 2
  spline S194 degree 2 poles (15.588, 28.1779) (15.588, 28) (15.5164, 27.7333) (15.4077, 27.5875) knots 0 0 0 1 2 2 2
  spline S195 degree 2 poles (15.4077, 27.5875) (15.2817, 27.4196) (14.8914, 27.2566) (14.6296, 27.2566) knots 0 0 0 1 2 2 2
  spline S196 degree 2 poles (14.6123, 27.6715) (14.8, 27.6715) (15.0545, 27.7703) (15.1434, 27.879) knots 0 0 0 1 2 2 2
  spline S197 degree 2 poles (15.1434, 27.879) (15.2076, 27.9605) (15.2496, 28.1631) (15.2496, 28.2693) knots 0 0 0 1 2 2 2
  spline S198 degree 2 poles (15.2496, 28.2693) (15.2496, 28.4125) (15.1631, 28.6818) (15.0816, 28.8127) knots 0 0 0 1 2 2 2
  spline S199 degree 2 poles (15.0816, 28.8127) (15.0372, 28.8151) (14.9532, 28.8201) (14.889, 28.8201) knots 0 0 0 1 2 2 2
  spline S200 degree 2 poles (14.889, 28.8201) (14.5728, 28.8201) (14.185, 28.6966) (14.0837, 28.6027) knots 0 0 0 1 2 2 2
  spline S201 degree 2 poles (14.0837, 28.6027) (13.9874, 28.5163) (13.9108, 28.3285) (13.9108, 28.2223) knots 0 0 0 1 2 2 2
  spline S202 degree 2 poles (13.9108, 28.2223) (13.9108, 27.9753) (14.2616, 27.6715) (14.6123, 27.6715) knots 0 0 0 1 2 2 2
  point P0 (0, 18.8295)
  constraints: 2 other
extrude "label" cut sketch "label_sketch" against normal blind 1
sketch "Sketch12" plane through (0, 0, 34) normal (0, 0, 1) x (1, 0, 0)
  circle A0 centre (-12.5, 37.5) radius 3.25
  circle A1 centre (-12.25, -12.5) radius 3.25
  circle A2 centre (-37.5, -12.5795) radius 3.25
  circle A3 centre (-37.5, 37.5) radius 3.25
  point P0 (0, 0)
  constraints: 4 centre point
hole "Hole2" at (-12.5, 37.5, 34) at (-37.5, 37.5, 34) at (-37.5, -12.5795, 34) at (-12.25, -12.5, 34) direction (0, 0, -1) diameter 6.5 end through all
hole "Hole3" at (-37.5, 37.5, 34) at (-12.5, 37.5, 34) at (-12.25, -12.5, 34) at (-37.5, -12.5795, 34) direction (0, 0, -1) diameter 10.5 depth 6 tip angle 118
hole "Hole4" at (-3.0004, 28.5366, 34) at (-3.0004, -3.4634, 34) at (-43.0004, 12.5366, 34) direction (0, 0, -1) diameter 6.5 end through all
equation "\"d31\" = d30"
equation "\"d62\" = d61"
equation "\"d63\" = d61"
body "Solid3"
